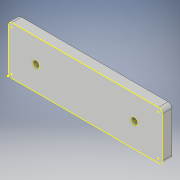
# Autodesk Inventor part: BasePatasVTOL
Saved by Autodesk Inventor 2019 (Build 230136000, 136)
## iProperties
Created: 2019-04-08
Part Number: BasePatasVTOL
Material: Generic
Document SubType Name: Modeling
Designer: Kenny
Density: 1 g/cm^3
Appearance: Default
Author: Kenny
Autodesk Inventor part; units mm, degrees
ref_plane "YZ Plane" through (0, 0, 0) normal (1, 0, 0) x (0, 1, 0)
ref_plane "XZ Plane" through (0, 0, 0) normal (0, 1, 0) x (-1, 0, 0)
ref_plane "XY Plane" through (0, 0, 0) normal (0, 0, 1) x (1, 0, 0)
sketch "Sketch1" plane through (0, 0, 0) normal (0, 0, 1) x (1, 0, 0)
  line L0 (0, 0) -> (80, 0)
  line L1 (80, 0) -> (80, 25)
  line L2 (80, 25) -> (0, 25)
  line L3 (0, 25) -> (0, 0)
  point P0 (14.5, 12.5)
  point P1 (65.5, 12.5)
  dimension "d0" = 80
  dimension "d1" = 25
  dimension "d2" = 12.5
  dimension "d3" = 14.5
  dimension "d4" = 51
  constraints: 8 end point, 2 parallel, 1 horizontal, 1 horizontal alignment, 1 perpendicular
  measures "d0" distance of L2.end L1.end
  measures "d1" distance of L1.end L0.end
  measures "d2" distance from line of L0 point (14.5, 12.5)
  measures "d3" distance from line of L3 point (14.5, 12.5)
  measures "d4" distance of point (65.5, 12.5) point (14.5, 12.5)
extrude "Extrusion1" add sketch "Sketch1" along normal blind 5
sketch "Sketch2" plane through (0, 0, 0) normal (0, 0, 1) x (1, 0, 0)
  line L0 (0, 0) -> (80, 0)
  line L1 (80, 0) -> (80, 25)
  line L2 (80, 25) -> (0, 25)
  line L3 (0, 25) -> (0, 0)
  point P0 (14.5, 12.5)
  point P1 (65.5, 12.5)
  dimension "d5" = 80
  dimension "d6" = 25
  dimension "d7" = 12.5
  dimension "d8" = 14.5
  dimension "d9" = 51
  constraints: 8 end point, 2 parallel, 1 horizontal, 1 horizontal alignment, 1 perpendicular
  measures "d5" distance of L2.end L1.end
  measures "d6" distance of L1.end L0.end
  measures "d7" distance from line of L0 point (14.5, 12.5)
  measures "d8" distance from line of L3 point (14.5, 12.5)
  measures "d9" distance of point (65.5, 12.5) point (14.5, 12.5)
hole "Hole1" at (14.5, 12.5, 0) at (65.5, 12.5, 0) direction (0, 0, 1) diameter 3.5 end through all
fillet "Fillet1" radius 2 4 edges at (0, 25, 2.5) (80, 25, 2.5) (80, 0, 2.5) (0, 0, 2.5)
sketch "Sketch3" plane through (0, 0, 5) normal (0, 0, 1) x (1, 0, 0)
  arc A0 (0, 2) -> (2, 0) centre (2, 2) ccw projected
  line L0 (2, 0) -> (78, 0) projected
  arc A1 (78, 0) -> (80, 2) centre (78, 2) ccw projected
  line L1 (80, 2) -> (80, 23) projected
  arc A2 (80, 23) -> (78, 25) centre (78, 23) ccw projected
  line L2 (78, 25) -> (2, 25) projected
  arc A3 (2, 25) -> (0, 23) centre (2, 23) ccw projected
  line L3 (0, 23) -> (0, 2) projected
  circle A4 centre (14.5, 12.5) radius 1.75 projected
  circle A5 centre (65.5, 12.5) radius 1.75 projected
  point P0 (0, 0)
body "Solid1"
